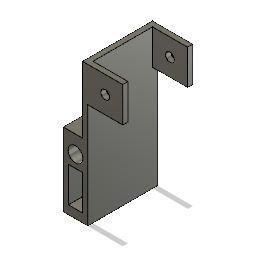
SliderMotor (Autodesk Fusion 360 design; units mm, degrees)
Autodesk Fusion 360 part; units mm, degrees
note: some values were not read from the file. Chosen so that the rebuilt part matches the saved one: which bodies a step acts on.
sketch "Sketch1" plane through (0, 0, 0) normal (0, 1, 0) x (1, 0, 0)
  line L0 (5, 20) -> (-5, 20)
  line L1 (-5, 20) -> (-5, -20)
  line L2 (-5, -20) -> (5, -20)
  line L3 (5, -20) -> (5, 20)
  line L4 (5, 20) -> (-5, -20) construction
  line L5 (-5, 20) -> (5, -20) construction
  line L6 (-5, -20) -> (-8, -20)
  line L7 (-8, -20) -> (-8, 20)
  line L8 (-8, 20) -> (-5, 20)
  line L9 (-5, 20) -> (-5, -20)
  line L10 (5, -20) -> (8, -20)
  line L11 (8, -20) -> (8, 20)
  line L12 (8, 20) -> (5, 20)
  line L13 (5, 20) -> (5, -20)
  dimension "d1" = 10
  dimension "d2" = 40
  dimension "d3" = 3
  dimension "d4" = 40
  dimension "d5" = 3
  dimension "d6" = 40
  constraint horizontal L0
  constraint perpendicular L0 L1
  constraint parallel L0 L2
  constraint parallel L1 L3
  constraint coincident L4 origin
  constraint coincident L5 origin
  constraint horizontal L6
  constraint vertical L7
  constraint horizontal L8
  constraint vertical L9
  constraint horizontal L10
  constraint vertical L11
  constraint horizontal L12
  constraint vertical L13
  measures "d1" distance of L1.end L2.end
  measures "d2" distance of L0.end L1.end
  measures "d3" distance of L1.end L6.end
  measures "d4" distance of L1.end L0.end
  measures "d5" distance of L2.end L10.end
  measures "d6" distance of L2.end L0.start
extrude "Extrude1" add sketch "Sketch1" along normal blind 80 contours L1 L6 L7 L8 L9 makes body 1
extrude "Extrude2" add sketch "Sketch1" along normal blind 80 separate body contours L3 L10 L11 L12 L13 makes body 2
extrude "Extrude3" add sketch "Sketch1" along normal blind 10 contours L0 L1 L2 L3 L9 L13 bodies 1 2
sketch "Sketch2" plane through (0, 0, 0) normal (0, 1, 0) x (1, 0, 0)
  line L0 (0, 0) -> (0, -8) construction
  line L1 (0, 0) -> (0, 8) construction
  circle A0 centre (0, -8) radius 1.5
  circle A1 centre (0, 8) radius 1.5
  dimension "d13" = 8
  dimension "d14" = 8
  dimension "d15" = 3
  dimension "d16" = 3
  constraint coincident L0.start L1.start
  constraint vertical L0
  constraint parallel L0 L1
  constraint coincident L0.end A0.centre
  constraint coincident L1.end A1.centre
  measures "d13" distance of L0.start L0.end
  measures "d14" distance of L0.start L1.end
  measures "d15" diameter of A0
  measures "d16" diameter of A1
extrude "Extrude4" cut sketch "Sketch2" along normal blind 10 contours A0 bodies 1
extrude "Extrude5" cut sketch "Sketch2" along normal blind 10 contours A1 bodies 1
extrude "Extrude6" cut sketch "Sketch1" along normal blind 10 contours L0 L1 L2 L3 L9 L13 bodies 1 makes body 3 at (-5, 26.6667, -6.6667)
extrude "Extrude7" add sketch "Sketch1" along normal blind 5 contours L0 L1 L2 L3 L9 L13 bodies 1 3
extrude "Extrude8" cut sketch "Sketch2" along normal blind 5 contours A0 bodies 1
extrude "Extrude9" cut sketch "Sketch2" along normal blind 5 contours A1 bodies 1
sketch "Sketch3" plane through (8, 0, 0) normal (1, 0, 0) x (0, 0, -1)
  line L0 (-20, 0) -> (20, 0)
  line L1 (20, 0) -> (20, 80)
  line L2 (20, 80) -> (-20, 80)
  line L3 (-20, 80) -> (-20, 0)
  line L4 (-20, 80) -> (20, 80)
  line L5 (20, 80) -> (20, 60)
  line L6 (20, 60) -> (-20, 60)
  line L7 (-20, 60) -> (-20, 80)
  dimension "d29" = 20
  constraint horizontal L4
  constraint vertical L5
  constraint horizontal L6
  constraint vertical L7
  constraint coincident L2.end L3.start
  measures "d29" distance of L2.end L6.end
extrude "Extrude10" add sketch "Sketch3" along normal blind 20 contours L1 L2 L3 L4 L5 L6 L7 bodies 1
sketch "Sketch4" plane through (28, 0, 0) normal (1, 0, 0) x (0, 0, -1)
  line L0 (-20, 60) -> (20, 60)
  line L1 (20, 60) -> (20, 80)
  line L2 (20, 80) -> (-20, 80)
  line L3 (-20, 80) -> (-20, 60)
  line L4 (17, 80) -> (-17, 80)
  line L5 (-17, 80) -> (-17, 60)
  line L6 (-17, 60) -> (17, 60)
  line L7 (17, 60) -> (17, 80)
  line L8 (17, 80) -> (-17, 60) construction
  line L9 (-17, 80) -> (17, 60) construction
  point P0 (0, 70)
  dimension "d32" = 34
  constraint horizontal L4
  constraint perpendicular L4 L5
  constraint parallel L4 L6
  constraint parallel L5 L7
  constraint coincident L8 P0
  constraint coincident L9 P0
  measures "d32" distance of L5.end L6.end
extrude "Extrude11" cut sketch "Sketch4" against normal blind 20 contours L0 L2 L4 L5 L6 L7 bodies 1
sketch "Sketch5" plane through (0, 0, -20) normal (0, 0, -1) x (-1, 0, 0)
  line L0 (-5, 5) -> (-5, 80)
  line L1 (-5, 80) -> (-28, 80)
  line L2 (-28, 80) -> (-28, 60)
  line L3 (-28, 60) -> (-8, 60)
  line L4 (-8, 60) -> (-8, 0)
  line L5 (-8, 0) -> (8, 0)
  line L6 (8, 0) -> (8, 80)
  line L7 (8, 80) -> (5, 80)
  line L8 (5, 80) -> (5, 5)
  line L9 (5, 5) -> (-5, 5)
  line L10 (-28, 60) -> (-8, 60) construction
  line L11 (-8, 60) -> (-8, 80) construction
  line L12 (-8, 80) -> (-28, 80) construction
  line L13 (-28, 80) -> (-28, 60) construction
  line L14 (-28, 60) -> (-8, 80) construction
  line L15 (-28, 80) -> (-8, 60) construction
  circle A0 centre (-18, 70) radius 2.5
  dimension "d35" = 20
  dimension "d36" = 5
  constraint horizontal L10
  constraint vertical L11
  constraint horizontal L12
  constraint vertical L13
  constraint coincident L1 L11.end
  constraint coincident L2.end L3.start
  constraint coincident L1.end L2.start
  constraint coincident L3.end L4.start
  constraint midpoint L15 A0.centre
  measures "d35" distance of L2.end L3.end
  measures "d36" diameter of A0
extrude "Extrude12" cut sketch "Sketch5" against normal blind 3 contours A0 bodies 1
sketch "Sketch6" plane through (0, 0, 20) normal (0, 0, 1) x (1, 0, 0)
  line L0 (-8, 0) -> (8, 0)
  line L1 (8, 0) -> (8, 60)
  line L2 (8, 60) -> (28, 60)
  line L3 (28, 60) -> (28, 80)
  line L4 (28, 80) -> (5, 80)
  line L5 (5, 80) -> (5, 5)
  line L6 (5, 5) -> (-5, 5)
  line L7 (-5, 5) -> (-5, 80)
  line L8 (-5, 80) -> (-8, 80)
  line L9 (-8, 80) -> (-8, 0)
  circle A0 centre (18, 70) radius 2.5
  line L10 (28, 60) -> (28, 80)
  line L11 (28, 80) -> (8, 80)
  line L12 (8, 80) -> (8, 60)
  line L13 (8, 60) -> (28, 60)
  circle A1 centre (18, 70) radius 2.5
  constraint concentric A0 A1
extrude "Extrude13" cut sketch "Sketch6" against normal blind 3 contours A0 A1 bodies 1
ref_plane "WorkPlane1" through (4, 0, 0) normal (1, 0, 0) x (0, 1, 0)
ref_plane "WorkPlane2" through (-4, 0, 0) normal (1, 0, 0) x (0, 1, 0)
ref_plane "WorkPlane3" through (5, 42.5, 0) normal (-1, 0, 0) x (0, 0, 1)
ref_plane "WorkPlane4" through (-5, 42.5, 0) normal (1, 0, 0) x (0, 0, -1)
split "Split1" by plane through (-5, 42.5, 0) normal (1, 0, 0) and through (5, 42.5, 0) normal (-1, 0, 0) and through (4, 0, 0) normal (1, 0, 0) and through (-4, 0, 0) normal (1, 0, 0) bodies 1 makes body 4 at (8, 20, 5.6667) makes body 5 at (-4.6667, 5, 6.6667) makes body 6 at (4.3333, 5, 6.6667) makes body 7 at (0.0374, 5, 16.4986)
move_body "Move1" bodies 1 to x (1, 0, 0) y (0, 1, 0) z (0, 0, 1) at (1, 0, 0)
move_body "Move2" bodies 4 to x (1, 0, 0) y (0, 1, 0) z (0, 0, 1) at (-1, 0, 0)
delete_body "RemoveBody1" bodies 5
delete_body "RemoveBody2" bodies 6
combine "Combine1" operation add target body 1 tool bodies 4 7
sketch "Sketch7" plane through (0, 0, 20) normal (0, 0, 1) x (1, 0, 0)
  circle A0 centre (17, 70) radius 2.5
  line L0 (-4, 5) -> (-4, 80)
  line L1 (-4, 80) -> (-7, 80)
  line L2 (-7, 80) -> (-7, 0)
  line L3 (-7, 0) -> (7, 0)
  line L4 (7, 0) -> (7, 60)
  line L5 (7, 60) -> (27, 60)
  line L6 (27, 60) -> (27, 80)
  line L7 (27, 80) -> (4, 80)
  line L8 (4, 80) -> (4, 5)
  line L9 (4, 5) -> (-4, 5)
sketch "Sketch8" plane through (0, 0, 20) normal (0, 0, 1) x (1, 0, 0)
  line L0 (-4, 5) -> (-4, 40) construction
  line L1 (-4, 40) -> (-4, 32) construction
  line L2 (-4, 32) -> (-4, 42) construction
  line L3 (-4, 32) -> (4, 32) construction
  circle A0 centre (0, 32) radius 4.25
  line L4 (-4, 5) -> (4, 5)
  line L5 (4, 5) -> (4, 42)
  line L6 (4, 42) -> (-4, 42)
  line L7 (-4, 42) -> (-4, 5)
  line L8 (-4, 5) -> (4, 5)
  line L9 (4, 5) -> (4, 25)
  line L10 (4, 25) -> (-4, 25)
  line L11 (-4, 25) -> (-4, 5)
  dimension "d45" = 35
  dimension "d46" = 8
  dimension "d47" = 10
  dimension "d48" = 8.5
  dimension "d49" = 8
  dimension "d50" = 20
  constraint vertical L0
  constraint parallel L0 L1
  constraint parallel L1 L2
  constraint perpendicular L2 L3
  constraint midpoint L3 A0.centre
  constraint horizontal L4
  constraint vertical L5
  constraint horizontal L6
  constraint vertical L7
  constraint horizontal L8
  constraint vertical L9
  constraint horizontal L10
  constraint vertical L11
  measures "d45" distance of L0.start L0.end
  measures "d46" distance of L0.end L1.end
  measures "d47" distance of L1.end L2.end
  measures "d48" diameter of A0
  measures "d49" distance of L0.start L4.end
  measures "d50" distance of L0.start L10.end
extrude "Extrude14" add sketch "Sketch8" against normal blind 40 contours A0 L5 L7 | A0 L5 L6 L7 | A0 L5 L7 L10 bodies 1
extrude "Extrude15" cut sketch "Sketch8" against normal blind 40 contours A0 L5 L7 bodies 1
extrude "Extrude16" cut sketch "Sketch8" against normal blind 40 contours A0 L5 | A0 L7 bodies 1
ref_plane "WorkPlane5" through (0, 42, 0) normal (0, 1, 0) x (1, 0, 0)
split "Split2" by plane through (0, 42, 0) normal (0, 1, 0) bodies 1 makes body 8 at (4, 54.6667, 6.6667) makes body 9 at (-4, 54.6667, -6.6667)
delete_body "RemoveBody3" bodies 9
combine "Combine2" operation add target body 1 tool bodies 8
